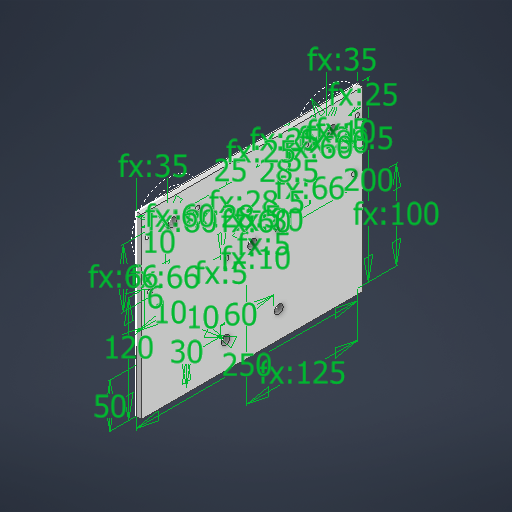
# Autodesk Inventor part: test_rig_plate
Saved by Autodesk Inventor 2027.1 (Build 311270010, 270A)
## iProperties
Created: 2026-09-04
Part Number: test_rig_plate
Material: Generic
Document SubType Name: Modeling
Designer: ajrcr
Density: 1 g/cm^3
Appearance: Default
Author: ajrcr
Autodesk Inventor part; units mm, degrees
ref_plane "YZ Plane" through (0, 0, 0) normal (1, 0, 0) x (0, 1, 0)
ref_plane "XZ Plane" through (0, 0, 0) normal (0, 1, 0) x (-1, 0, 0)
ref_plane "XY Plane" through (0, 0, 0) normal (0, 0, 1) x (1, 0, 0)
sketch "Sketch1" plane through (0, 0, 0) normal (1, 0, 0) x (0, 1, 0)
  line L0 (100, 125) -> (-100, 125)
  line L1 (-100, 125) -> (-100, -125)
  line L2 (-100, -125) -> (100, -125)
  line L3 (100, -125) -> (100, 125)
  circle A0 centre (75, 90) radius 5
  circle A1 centre (75, -90) radius 5
  circle A2 centre (9, 0) radius 5
  line L4 (100, 0) -> (-100, 0) construction
  line L5 (0, 125) -> (0, -125) construction
  circle A3 centre (-70, 30) radius 5
  line L6 (-50, 125) -> (-50, -125) construction
  circle A4 centre (75, 90) radius 30 construction
  circle A5 centre (75, -90) radius 30 construction
  circle A6 centre (9, 0) radius 30 construction
  line L7 (45, 125) -> (45, -125) construction
  line L8 (39, 125) -> (39, -125) construction
  circle A7 centre (9, 0) radius 40 construction
  circle A8 centre (75, 90) radius 40 construction
  circle A9 centre (75, -90) radius 40 construction
  circle A10 centre (-70, -30) radius 5
  circle A11 centre (20, 115) radius 3
  circle A12 centre (20, -115) radius 3
  circle A13 centre (75, -61.5) radius 2.5
  circle A14 centre (75, -118.5) radius 2.5
  circle A15 centre (75, 61.5) radius 2.5
  circle A16 centre (75, 118.5) radius 2.5
  circle A17 centre (9, -28.5) radius 2.5
  circle A18 centre (9, 28.5) radius 2.5
  point P0 (0, 0)
  dimension "plate_height" = 200
  dimension "plate_width" = 250
  dimension "d16" = 125
  dimension "d17" = 100
  dimension "axle_diam" = 10
  dimension "d19" = 10
  dimension "d20" = 10
  dimension "d21" = 35
  dimension "d22" = 35
  dimension "upper_wheel_height" = 25
  dimension "d24" = 25
  dimension "d25" = 66
  dimension "bracket_hole_diam" = 10
  dimension "bracket_hole_height" = 30
  dimension "bracket_height" = 50
  dimension "d29" = 60
  dimension "d30" = 60
  dimension "d31" = 60
  dimension "d32" = 80
  dimension "d33" = 80
  dimension "d34" = 80
  dimension "bracket_hole_spacing" = 60
  dimension "adj_thread_diam" = 6
  dimension "adj_thread_left" = 10
  dimension "adj_thread_bottom" = 120
  dimension "bearing_bracket_bolt" = 5
  dimension "d40" = 5
  dimension "d41" = 28.5
  dimension "d42" = 28.5
  dimension "d43" = 25
  dimension "d44" = 25
  dimension "d45" = 5
  dimension "d46" = 5
  dimension "d47" = 28.5
  dimension "d48" = 28.5
  dimension "d49" = 66
  dimension "d50" = 66
  constraints: 19 centre point, 18 end point, 7 point on line, 6 coincident, 4 midpoint, 4 symmetric about line, 3 perpendicular, 2 parallel, 2 tangent, 1 horizontal, 1 vertical, 4 other
  measures "plate_height" distance of L2.end L1.end
  measures "plate_width" distance of L1.end L0.end
  measures "d16" distance from line of point (0, 0) L2
  measures "d17" distance from line of point (0, 0) L1
  measures "axle_diam" diameter of A0
  measures "d19" diameter of A1
  measures "d20" diameter of A2
  measures "d21" distance from line of A0.centre L0
  measures "d22" distance from line of L2 A1.centre
  measures "upper_wheel_height" distance from line of A0.centre L3
  measures "d24" distance from line of L3 A1.centre
  measures "d25" horizontal distance of A2.centre A0.centre
  measures "bracket_hole_diam" diameter of A3
  measures "bracket_hole_height" distance from line of A3.centre L1
  measures "bracket_height" distance between parallel lines of L1 L6
  measures "d29" diameter of A4
  measures "d30" diameter of A5
  measures "d31" diameter of A6
  measures "d32" diameter of A7
  measures "d33" diameter of A8
  measures "d34" diameter of A9
  measures "bracket_hole_spacing" distance of A3.centre A10.centre
  measures "adj_thread_diam" diameter of A11
  measures "adj_thread_left" distance from line of A11.centre L0
  measures "adj_thread_bottom" distance from line of A11.centre L1
  measures "bearing_bracket_bolt" diameter of A13
  measures "d40" diameter of A14
  measures "d41" distance of A13.centre A1.centre
  measures "d42" distance of A14.centre A1.centre
  measures "d43" distance from line of L3 A13.centre
  measures "d44" distance from line of L3 A14.centre
  measures "d45" diameter of A17
  measures "d46" diameter of A18
  measures "d47" distance of A18.centre A2.centre
  measures "d48" distance of A17.centre A2.centre
  measures "d49" horizontal distance of A0.centre A18.centre
  measures "d50" horizontal distance of A13.centre A17.centre
extrude "Extrusion1" add sketch "Sketch1" along normal blind 6
equation "\"d16\" = 0.5 * plate_width"
equation "\"d17\" = 0.5 * plate_height"
equation "\"d19\" = axle_diam"
equation "\"d20\" = axle_diam"
equation "\"d21\" = -0.5 * upper_wheel_pitch + 0.5 * plate_width"
equation "\"d22\" = -0.5 * upper_wheel_pitch + 0.5 * plate_width"
equation "\"d24\" = upper_wheel_height"
equation "\"d29\" = wheel_diam"
equation "\"d30\" = wheel_diam"
equation "\"d31\" = wheel_diam"
equation "\"d32\" = wheel_flange_diam"
equation "\"d33\" = wheel_flange_diam"
equation "\"d34\" = wheel_flange_diam"
equation "\"d40\" = bearing_bracket_bolt"
equation "\"d42\" = d41"
equation "\"d43\" = upper_wheel_height"
equation "\"d44\" = upper_wheel_height"
equation "\"d45\" = bearing_bracket_bolt"
equation "\"d46\" = bearing_bracket_bolt"
equation "\"d47\" = d41"
equation "\"d48\" = d41"
equation "\"d49\" = d25"
equation "\"d50\" = d49"
equation "\"wheel_diam\" = 60"
equation "\"wheel_flange_diam\" = 80"
equation "\"upper_wheel_pitch\" = 180"
body "Solid1"
